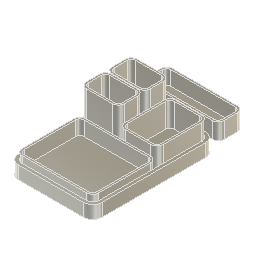
Модный органайзер от ПЭС (Autodesk Fusion 360 design; units mm, degrees)
Autodesk Fusion 360 part; units mm, degrees
sketch "Sketch1" plane through (0, 0, 0) normal (0, 0, 1) x (1, 0, 0)
  line L0 (50, 90) -> (-50, 90)
  line L1 (-65, 75) -> (-65, -85)
  line L2 (-50, -100) -> (50, -100)
  line L3 (65, -85) -> (65, 75)
  arc A0 (65, 75) -> (50, 90) centre (50, 75) ccw
  arc A1 (-50, 90) -> (-65, 75) centre (-50, 75) ccw
  arc A2 (-65, -85) -> (-50, -100) centre (-50, -85) ccw
  arc A3 (50, -100) -> (65, -85) centre (50, -85) ccw
  line L4 (50, 85) -> (-50, 85)
  arc A4 (-50, 85) -> (-60, 75) centre (-50, 75) ccw
  line L5 (-60, 75) -> (-60, -85)
  arc A5 (-60, -85) -> (-50, -95) centre (-50, -85) ccw
  line L6 (-50, -95) -> (50, -95)
  arc A6 (50, -95) -> (60, -85) centre (50, -85) ccw
  line L7 (60, -85) -> (60, 75)
  arc A7 (60, 75) -> (50, 85) centre (50, 75) ccw
  arc A8 (59.6, 75) -> (50, 84.6) centre (50, 75) ccw
  line L8 (50, 84.6) -> (10, 84.6)
  arc A9 (10, 84.6) -> (0.4, 75) centre (10, 75) ccw
  line L9 (0.4, 75) -> (0.4, 55)
  line L10 (59.6, 55) -> (59.6, 75)
  line L11 (59.6, 55) -> (59.6, 75)
  arc A10 (59.6, 75) -> (50, 84.6) centre (50, 75) ccw
  line L12 (50, 84.6) -> (10, 84.6)
  arc A11 (10, 84.6) -> (0.4, 75) centre (10, 75) ccw
  line L13 (0.4, 75) -> (0.4, 55)
  line L14 (-49.9597, 45.4624) -> (-10.0026, 45.4)
  arc A12 (-59.5415, 55.0026) -> (-49.9597, 45.4624) centre (-49.9417, 55.0623) ccw
  line L15 (-59.6, 74.9952) -> (-59.5415, 55.0026)
  arc A13 (-50, 84.6) -> (-59.6, 74.9952) centre (-50, 75) ccw
  line L16 (-10, 84.6) -> (-50, 84.6)
  arc A14 (-0.4, 75) -> (-10, 84.6) centre (-10, 75) ccw
  line L17 (-0.4, 55) -> (-0.4, 75)
  arc A15 (-10.0026, 45.4) -> (-0.4, 55) centre (-10, 55) ccw
  line L18 (10, 5.4) -> (50, 5.4)
  arc A16 (0.4, 15) -> (10, 5.4) centre (10, 15) ccw
  line L19 (0.4, 35) -> (0.4, 15)
  line L20 (59.6, 15) -> (59.6, 35)
  arc A17 (50, 5.4) -> (59.6, 15) centre (50, 15) ccw
  line L21 (-50, 5.4) -> (-10, 5.4)
  arc A18 (-59.6, 15) -> (-50, 5.4) centre (-50, 15) ccw
  line L22 (-59.6, 35) -> (-59.6, 15)
  arc A19 (-50, 44.6) -> (-59.6, 35) centre (-50, 35) ccw
  line L23 (-10, 44.6) -> (-50, 44.6)
  arc A20 (-0.4, 35) -> (-10, 44.6) centre (-10, 35) ccw
  line L24 (-0.4, 15) -> (-0.4, 35)
  arc A21 (-10, 5.4) -> (-0.4, 15) centre (-10, 15) ccw
  line L25 (-50, -94.6) -> (50, -94.6)
  arc A22 (-59.6, -85) -> (-50, -94.6) centre (-50, -85) ccw
  line L26 (-59.6, -5) -> (-59.6, -85)
  arc A23 (-50, 4.6) -> (-59.6, -5) centre (-50, -5) ccw
  line L27 (50, 4.6) -> (-50, 4.6)
  arc A24 (59.6, -5) -> (50, 4.6) centre (50, -5) ccw
  line L28 (59.6, -85) -> (59.6, -5)
  arc A25 (50, -94.6) -> (59.6, -85) centre (50, -85) ccw
  arc A26 (-50, 1.6) -> (-56.6, -5) centre (-50, -5) ccw
  line L29 (-56.6, -5) -> (-56.6, -85)
  arc A27 (-56.6, -85) -> (-50, -91.6) centre (-50, -85) ccw
  line L30 (-50, -91.6) -> (50, -91.6)
  arc A28 (50, -91.6) -> (56.6, -85) centre (50, -85) ccw
  line L31 (56.6, -85) -> (56.6, -5)
  arc A29 (56.6, -5) -> (50, 1.6) centre (50, -5) ccw
  line L32 (50, 1.6) -> (-50, 1.6)
  arc A30 (-3.4, 75) -> (-10, 81.6) centre (-10, 75) ccw
  line L33 (-10, 81.6) -> (-50, 81.6)
  arc A31 (-50, 81.6) -> (-56.6, 75) centre (-50, 75) ccw
  line L34 (-56.6, 75) -> (-56.5417, 55.0693)
  arc A32 (-56.5417, 55.0693) -> (-49.9494, 48.4623) centre (-49.9417, 55.0623) ccw
  line L35 (-49.9494, 48.4623) -> (-10, 48.4)
  arc A33 (-10, 48.4) -> (-3.4, 55) centre (-10, 55) ccw
  line L36 (-3.4, 55) -> (-3.4, 75)
  arc A34 (-50, 41.6) -> (-56.6, 35) centre (-50, 35) ccw
  line L37 (-56.6, 35) -> (-56.6, 15)
  arc A35 (-56.6, 15) -> (-50, 8.4) centre (-50, 15) ccw
  line L38 (-50, 8.4) -> (-10, 8.4)
  arc A36 (-10, 8.4) -> (-3.4, 15) centre (-10, 15) ccw
  line L39 (-3.4, 15) -> (-3.4, 35)
  arc A37 (-3.4, 35) -> (-10, 41.6) centre (-10, 35) ccw
  line L40 (-10, 41.6) -> (-50, 41.6)
  line L41 (0.4, 35) -> (0.4, 55)
  line L42 (59.6, 55) -> (59.6, 35)
  line L43 (56.6, 55) -> (56.6, 35)
  line L44 (56.6, 15) -> (56.6, 35)
  arc A38 (50, 8.4) -> (56.6, 15) centre (50, 15) ccw
  line L45 (10, 8.4) -> (50, 8.4)
  arc A39 (3.4, 15) -> (10, 8.4) centre (10, 15) ccw
  line L46 (3.4, 35) -> (3.4, 15)
  line L47 (3.4, 35) -> (3.4, 55)
  line L48 (3.4, 75) -> (3.4, 55)
  arc A40 (10, 81.6) -> (3.4, 75) centre (10, 75) ccw
  line L49 (50, 81.6) -> (10, 81.6)
  arc A41 (56.6, 75) -> (50, 81.6) centre (50, 75) ccw
  line L50 (56.6, 55) -> (56.6, 75)
  arc A42 (-59.5415, 110.0026) -> (-49.9597, 100.4624) centre (-49.9417, 110.0623) ccw
  arc A43 (-50, 139.6) -> (-59.6, 129.9952) centre (-50, 130) ccw
  line L51 (-59.6, 129.9952) -> (-59.5415, 110.0026)
  line L52 (-56.6, 130) -> (-56.5417, 110.0693)
  arc A44 (-50, 136.6) -> (-56.6, 130) centre (-50, 130) ccw
  line L53 (50, 139.6) -> (-50, 139.6)
  line L54 (50, 136.6) -> (-50, 136.6)
  arc A45 (-56.5417, 110.0693) -> (-49.9494, 103.4623) centre (-49.9417, 110.0623) ccw
  line L55 (-49.9545, 103.4624) -> (-49.9494, 103.4623)
  arc A46 (50, 103.4) -> (56.6, 110) centre (50, 110) ccw
  arc A47 (49.9974, 100.4) -> (59.6, 110) centre (50, 110) ccw
  line L56 (59.6, 110) -> (59.6, 130)
  line L57 (56.6, 110) -> (56.6, 130)
  arc A48 (56.6, 130) -> (50, 136.6) centre (50, 130) ccw
  arc A49 (59.6, 130) -> (50, 139.6) centre (50, 130) ccw
  line L58 (50, 103.4) -> (-49.9545, 103.4624)
  line L59 (-49.9597, 100.4624) -> (49.9974, 100.4)
  point P0 (25, 40)
  dimension "d3" = 15
  dimension "d4" = -5
  dimension "d6" = 100
  dimension "d7" = 10
  dimension "d8" = 180
  dimension "d9" = 120
  dimension "d16" = -3
  dimension "d17" = -3
  dimension "d18" = -3
  dimension "d37" = -3
  constraint horizontal L0
  constraint perpendicular L0 L1
  constraint parallel L0 L2
  constraint parallel L1 L3
  constraint tangent L3 A0
  constraint tangent L0 A0
  constraint tangent L0 A1
  constraint tangent L1 A1
  constraint equal A0 A1
  constraint tangent L1 A2
  constraint tangent L2 A2
  constraint equal A0 A2
  constraint tangent L2 A3
  constraint tangent L3 A3
  constraint equal A0 A3
  constraint coincident A2.centre A5.centre
  constraint coincident A3.centre A6.centre
  constraint parallel L9 L41
  constraint parallel L20 L42
  constraint concentric A48 A49
  constraint concentric A46 A47
  constraint tangent L57 A48
  constraint tangent L54 A48
  constraint tangent A46 L57
  constraint concentric A43 A44
  constraint concentric A42 A45
  constraint tangent A44 L54
  constraint coincident A45 L55.start
  measures "d3" radius of A0
  measures "d6" distance of A5.end L6.end
  measures "d7" radius of A5
  measures "d8" distance of L4 L6
  measures "d9" distance of L5 L7
extrude "Extrude1" add sketch "Sketch1" along normal blind 4 contours L0 L1 L2 L3 A0 A1 A2 A3 | L4 A4 L5 A5 L6 A6 L7 A7 | A8 L8 A9 L9 L10 L11 A10 L12 A11 L13 L18 A16 L19 L20 A17 L41 L42 | L14 A12 L15 A13 L16 A14 L17 A15 | L21 A18 L22 A19 L23 A20 L24 A21 | L25 A22 L26 A23 L27 A24 L28 A25 | A26 L29 A27 L30 A28 L31 A29 L32 | A30 L33 A31 L34 A32 L35 A33 L36 | A34 L37 A35 L38 A36 L39 A37 L40 | L43 L44 A38 L45 A39 L46 L47 L48 A40 L49 A41 L50 makes body 1
extrude "Extrude2" add sketch "Sketch1" along normal blind 20 contours L0 L1 L2 L3 A0 A1 A2 A3 bodies 1
extrude "Extrude3" add sketch "Sketch1" along normal blind 7.5 and the other way blind -4.5 separate body contours A8 L8 A9 L9 L10 L11 A10 L12 A11 L13 L18 A16 L19 L20 A17 L41 L42 | L14 A12 L15 A13 L16 A14 L17 A15 | L21 A18 L22 A19 L23 A20 L24 A21 | L25 A22 L26 A23 L27 A24 L28 A25 | A26 L29 A27 L30 A28 L31 A29 L32 | A30 L33 A31 L34 A32 L35 A33 L36 | A34 L37 A35 L38 A36 L39 A37 L40 | L43 L44 A38 L45 A39 L46 L47 L48 A40 L49 A41 L50 makes body 2 at (-23.3333, 31.5333, 4.5) makes body 3 at (-23.3208, 58.4875, 4.5) makes body 4 at (20.1333, 35, 4.5) makes body 5 at (-16.6667, -28.4667, 4.5)
extrude "Extrude8" add sketch "Sketch1" along normal blind 30 and the other way blind -5 contours L14 A12 L15 A13 L16 A14 L17 A15 | L21 A18 L22 A19 L23 A20 L24 A21 bodies 2 3
extrude "Extrude9" add sketch "Sketch1" along normal blind 30 and the other way blind -5 contours A8 L8 A9 L9 L10 L11 A10 L12 A11 L13 L18 A16 L19 L20 A17 L41 L42 bodies 4
extrude "Extrude10" add sketch "Sketch1" along normal blind 30 and the other way blind -5 contours L25 A22 L26 A23 L27 A24 L28 A25 bodies 5
extrude "Extrude11" add sketch "Sketch1" along normal blind 7.5 and the other way blind -4.5 separate body contours A42 A43 L51 L53 A47 L56 A49 L59 | L52 A44 L54 A45 L55 A46 L57 A48 L58 makes body 6
extrude "Extrude12" add sketch "Sketch1" along normal blind 30 and the other way blind -5 contours A42 A43 L51 L53 A47 L56 A49 L59 bodies 6
extrude "Extrude13" add 2 faces at (-23.3333, 42.6, 30) (-36.6372, 46.4416, 30) along direction (0, 0, 1) blind 40 on bodies 2 3 bodies 2 3
extrude "Extrude14" add 1 faces at (57.6, 55, 30) along direction (0, 0, 1) blind 15 on bodies 4 bodies 4
